J6 (Autodesk Fusion 360 design; units mm, degrees)
part number: 2026-05-31-09-53-49-850
Autodesk Fusion 360 part; units mm, degrees
sketch "Sketch1" plane through (0, 0, 0) normal (0, 0, 1) x (1, 0, 0)
  line L0 (0, 0) -> (60, 0)
  circle A0 centre (5.2335, 14.8997) radius 4
  circle A1 centre (15, 15) radius 4
  circle A2 centre (45, 15) radius 4
  circle A3 centre (55, 15) radius 4
  circle A4 centre (5.2335, 4.9255) radius 4
  circle A5 centre (55, 5) radius 4
  line L1 (0, 0) -> (60, 0)
  line L2 (60, 0) -> (60, 40)
  line L3 (60, 40) -> (0, 40)
  line L4 (0, 40) -> (0, 0)
  circle A6 centre (30, 30) radius 4
  circle A7 centre (15, 5) radius 1.25
  circle A8 centre (45, 5) radius 1.25
  circle A9 centre (15, 30) radius 1.25
  circle A10 centre (45, 30) radius 1.25
  dimension "d1" = 60
  dimension "d3" = 8
  dimension "d4" = 8
  dimension "d5" = 8
  dimension "d6" = 8
  dimension "d7" = 8
  dimension "d8" = 8
  dimension "d9" = 40
  dimension "d10" = 8
  dimension "d11" = 2.5
  dimension "d12" = 2.5
  dimension "d13" = 2.5
  dimension "d14" = 2.5
  constraint horizontal L0
  constraint coincident L0.start L1.start
  constraint horizontal L1
  constraint vertical L2
  constraint horizontal L3
  constraint vertical L4
  measures "d1" distance of L0.start L0.end
  measures "d3" diameter of A0
  measures "d4" diameter of A1
  measures "d5" diameter of A2
  measures "d6" diameter of A3
  measures "d7" diameter of A4
  measures "d8" diameter of A5
  measures "d9" distance of L0.start L3.end
  measures "d10" diameter of A6
  measures "d11" diameter of A7
  measures "d12" diameter of A8
  measures "d13" diameter of A9
  measures "d14" diameter of A10
extrude "Extrude1" add sketch "Sketch1" along normal blind 5 makes body 1
copy_body "CopyPasteBodies1" bodies 1 makes body 2
move_body "Move1" bodies 2 to x (0.819152, 0, 0.573576) y (0, 1, 0) z (-0.573576, 0, 0.819152) at (-49.0945, 0, -34.1493)
extrude "Extrude2" add 1 faces at (0, 26.6667, 1.6667) along direction (-1, 0, 0) blind 3 on bodies 1 bodies 1 2
sketch "Sketch2" plane through (-2.9746, 0, 4.2481) normal (-0.573576, 0, 0.819152) x (0, -1, 0)
  circle A0 centre (-4.9255, -54.5696) radius 4
  circle A1 centre (-30, -29.8031) radius 4
  circle A2 centre (-15, -44.8031) radius 4
  circle A3 centre (-5, -4.8031) radius 4
  circle A4 centre (-15, -14.8031) radius 4
  circle A5 centre (-15, -4.8031) radius 4
  circle A6 centre (-5, -44.8031) radius 1.25
  circle A7 centre (-30, -44.8031) radius 1.25
  circle A8 centre (-14.8997, -54.5696) radius 4
  circle A9 centre (-30, -14.8031) radius 1.25
  circle A10 centre (-5, -14.8031) radius 1.25
  line L0 (0, -0.0311) -> (-40, -0.0311)
  line L1 (-40, -0.0311) -> (-40, -59.8031)
  line L2 (-40, -59.8031) -> (0, -59.8031)
  line L3 (0, -59.8031) -> (0, -0.0311)
  circle A11 centre (-15, -4.8031) radius 4
  circle A12 centre (-5, -4.8031) radius 4
  dimension "d19" = 8
  dimension "d20" = 8
  constraint concentric A5 A11
  constraint concentric A3 A12
  measures "d19" diameter of A11
  measures "d20" diameter of A12
extrude "Extrude3" cut sketch "Sketch2" against normal blind 10 contours A3 A12 | A5 A11 bodies 1
sketch "Sketch3" plane through (0, 0, 5) normal (0, 0, 1) x (-1, 0, 0)
  circle A0 centre (-45, -5) radius 1.25
  circle A1 centre (-45, -30) radius 1.25
  circle A2 centre (-5.2335, -14.8997) radius 4
  circle A3 centre (-15, -30) radius 1.25
  circle A4 centre (-15, -5) radius 1.25
  circle A5 centre (-55, -15) radius 4
  circle A6 centre (-45, -15) radius 4
  circle A7 centre (-55, -5) radius 4
  circle A8 centre (-15, -15) radius 4
  line L0 (3, 0) -> (-60, 0)
  line L1 (-60, 0) -> (-60, -40)
  line L2 (-60, -40) -> (3, -40)
  line L3 (3, -40) -> (3, 0)
  circle A9 centre (-30, -30) radius 4
  circle A10 centre (-5.2335, -4.9255) radius 4
sketch "Sketch4" plane through (0, 0, 5) normal (0, 0, 1) x (-1, 0, 0)
sketch "Sketch5" plane through (-2.9746, 0, 4.2481) normal (-0.573576, 0, 0.819152) x (0, -1, 0)
  circle A0 centre (-4.9255, -54.5696) radius 4
  circle A1 centre (-30, -29.8031) radius 4
  circle A2 centre (-15, -44.8031) radius 4
  circle A3 centre (-5, -4.8031) radius 4
  circle A4 centre (-15, -14.8031) radius 4
  circle A5 centre (-15, -4.8031) radius 4
  circle A6 centre (-5, -44.8031) radius 1.25
  circle A7 centre (-30, -44.8031) radius 1.25
  circle A8 centre (-14.8997, -54.5696) radius 4
  circle A9 centre (-30, -14.8031) radius 1.25
  circle A10 centre (-5, -14.8031) radius 1.25
  line L0 (0, -0.0311) -> (-40, -0.0311)
  line L1 (-40, -0.0311) -> (-40, -59.8031)
  line L2 (-40, -59.8031) -> (0, -59.8031)
  line L3 (0, -59.8031) -> (0, -0.0311)
sketch "Sketch6" plane through (-2.9746, 0, 4.2481) normal (-0.573576, 0, 0.819152) x (0, -1, 0)
fillet "Fillet1" radius 4.5 1 edges at (-3, 20, 5) on bodies 1
sketch "Sketch7" plane through (-2.9746, 0, 4.2481) normal (-0.573576, 0, 0.819152) x (0, -1, 0)
  circle A0 centre (-35, -45) radius 1.25
  circle A1 centre (-35, -15) radius 1.25
  dimension "d25" = 2.5
  dimension "d26" = 2.5
  measures "d25" diameter of A0
  measures "d26" diameter of A1
extrude "Extrude4" cut sketch "Sketch7" against normal blind 20 bodies 1
sketch "Sketch8" plane through (0, 0, 5) normal (0, 0, 1) x (-1, 0, 0)
  circle A0 centre (-45, -35) radius 1.25
  circle A1 centre (-15, -35) radius 1.25
  dimension "d29" = 2.5
  dimension "d30" = 2.5
  measures "d29" diameter of A0
  measures "d30" diameter of A1
extrude "Extrude5" cut sketch "Sketch8" against normal blind 20 bodies 1
sketch "Sketch9" plane through (-2.9746, 0, 4.2481) normal (-0.573576, 0, 0.819152) x (0, -1, 0)
